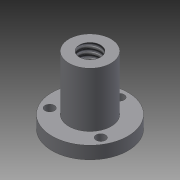
# Autodesk Inventor part: Lead_Screw_Flange_Nut
Saved by Autodesk Inventor 2015 (Build 190159000, 159)
## iProperties
Created: 2014-12-22
Part Number: Lead_Screw_Flange_Nut
Material: Generic
Document SubType Name: Modeling
Designer: Drew
Density: 1 g/cm^3
Appearance: Default
Author: Drew
Autodesk Inventor part; units mm, degrees
ref_plane "YZ Plane" through (0, 0, 0) normal (1, 0, 0) x (0, 1, 0)
ref_plane "XZ Plane" through (0, 0, 0) normal (0, 1, 0) x (-1, 0, 0)
ref_plane "XY Plane" through (0, 0, 0) normal (0, 0, 1) x (1, 0, 0)
sketch "Sketch1" plane through (0, 0, 0) normal (1, 0, 0) x (0, 1, 0)
  line L0 (0, 0) -> (25.4, 0)
  line L1 (25.4, 0) -> (25.4, -7.9375)
  line L2 (25.4, -7.9375) -> (4.7752, -7.9375)
  line L3 (4.7752, -7.9375) -> (4.7752, -14.2875)
  line L4 (4.7752, -14.2875) -> (0, -14.2875)
  line L5 (0, -14.2875) -> (0, 0)
  dimension "d0" = 25.4
  dimension "d1" = 4.7752
  dimension "d2" = 7.9375
  dimension "d3" = 14.2875
  constraints: 12 end point, 5 perpendicular, 1 horizontal
  measures "d0" distance between parallel lines of L1 L5
  measures "d1" distance of L3.end L4.end
  measures "d2" distance of L0.end L1.end
  measures "d3" distance between parallel lines of L0 L4
revolve "Revolution1" add sketch "Sketch1" angle 360 about axis through (0, 0, 0) along (0, 1, 0)
hole "Hole1" at (0, 25.4, 0) direction (0, -1, 0) diameter 8.001 end through all thread size "TR10x2" class "7H" standard "ISO Metric Trapezoidal Threads"
sketch "Sketch2" plane through (0, 4.7752, 0) normal (0, 1, 0) x (1, 0, 0)
  circle A0 centre (0, 0) radius 11.1125
  line L0 (-9.6237, -5.5562) -> (0, 0)
  line L1 (0, 0) -> (9.6237, -5.5562)
  line L2 (0, 0) -> (0, 11.1125)
  point P0 (-9.6237, -5.5562)
  dimension "d16" = 120
  dimension "d17" = 120
  dimension "d18" = 22.225
  constraints: 6 end point, 4 point on circle, 2 coincident, 1 centre point, 1 vertical
  measures "d16" angle of L0 L2
  measures "d17" angle of L2 L1
  measures "d18" diameter of A0
hole "Hole2" at (0, 4.7752, -11.1125) at (-9.6237, 4.7752, 5.5562) at (9.6237, 4.7752, 5.5562) direction (0, -1, 0) diameter 3.556 end through all
body "Solid1"
